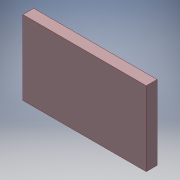
# Autodesk Inventor part: BMS_JBD-20-30s
Saved by Autodesk Inventor 2019.3 (Build 233278000, 278)
## iProperties
Created: 2019-03-05
Part Number: BMS_JBD-20-30s
Material: Generic
Document SubType Name: Modeling
Designer: eroldan
Density: 1 g/cm^3
Appearance: Default
Author: eroldan
Autodesk Inventor part; units mm, degrees
ref_plane "YZ Plane" through (0, 0, 0) normal (1, 0, 0) x (0, 1, 0)
ref_plane "XZ Plane" through (0, 0, 0) normal (0, 1, 0) x (-1, 0, 0)
ref_plane "XY Plane" through (0, 0, 0) normal (0, 0, 1) x (1, 0, 0)
sketch "Sketch1" plane through (0, 0, 0) normal (0, 0, 1) x (1, 0, 0)
  line L0 (-91.5, -55.25) -> (91.5, -55.25)
  line L1 (91.5, -55.25) -> (91.5, 55.25)
  line L2 (91.5, 55.25) -> (-91.5, 55.25)
  line L3 (-91.5, 55.25) -> (-91.5, -55.25)
  line L4 (-91.5, -55.25) -> (91.5, 55.25) construction
  line L5 (91.5, -55.25) -> (-91.5, 55.25) construction
  point P0 (0, 0)
  dimension "d0" = 183
  dimension "d1" = 110.5
  constraints: 12 end point, 2 midpoint, 2 parallel, 1 horizontal, 1 perpendicular
  measures "d0" distance of L2.end L1.end
  measures "d1" distance of L1.end L0.end
extrude "Extrusion1" add sketch "Sketch1" along normal blind 16
body "Solid1"
